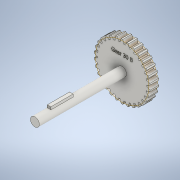
# Autodesk Inventor part: Spur_Gear12
Saved by Autodesk Inventor 2021 (Build 250183000, 183)
## iProperties
Created: 2021-04-10
Part Number: Spur_Gear12
Material: Steel
Document SubType Name: Modeling
Designer: Nabeel Azafer
Categories: <?xml version="1.0" encoding="UTF-16"?> <MemberInstance><Categories><FamilyTemplate><FamilyTemplateParameter ValueType="xs:double" Id="1" ObjectReferenceKey="da_z" ObjectType="kUserParameterObject"/><FamilyTemplateParameter ValueType="xs:double" Id="2" ObjectReferenceKey="da_b" ObjectType="kUserParameterObject"/><FamilyTemplateParameter ValueType="xs:double" Id="3" ObjectReferenceKey="da_beta" ObjectType="kUserParameterObject"/><FamilyTemplateParameter ValueType="xs:double" Id="4" ObjectReferenceKey="da_da" ObjectType="kUserParameterObject"/><FamilyTemplateParameter ValueType="xs:double" Id="5" ObjectReferenceKey="da_aw" ObjectType="kUserParameterObject"/><FamilyTemplateParameter ValueType="xs:string" Id="6" ObjectReferenceKey="EAIAABAAAACIAQAAAAAAAIAAAAAAAAAA" ObjectType="83910656" SubObjectId="SurfaceGeometry"/></FamilyTemplate><ParamToTemplateMap><ParamToTemplate CategoryParameter="//CategoryParameter[@InternalName='046C89C9-8512-4d59-83FE-43B91F4F132A']" TemplateParameter="1"/><ParamToTemplate CategoryParameter="//CategoryParameter[@InternalName='2552DF32-E462-4b46-AEBF-C6C7768E72AC']" TemplateParameter="2"/><ParamToTemplate CategoryParameter="//CategoryParameter[@InternalName='C9EE641D-15FC-4fae-A226-E94C4372FDD7']" TemplateParameter="3"/><ParamToTemplate><ParamToTemplate CategoryParameter="//CategoryParameter[@InternalName='00B6519A-459B-49c7-AD84-2E56D39A5744']" ConstantValue="0.000000"/></ParamToTemplate><ParamToTemplate><ParamToTemplate CategoryParameter="//CategoryParameter[@InternalName='04B31F0E-C7A6-4894-AA32-9629BEFACF47']" ConstantValue="0.800000"/></ParamToTemplate><ParamToTemplate><ParamToTemplate CategoryParameter="//CategoryParameter[@InternalName='43CBEC2E-7847-49e7-A936-2F7889FCB2D9']" ConstantValue="0.350000"/></ParamToTemplate><ParamToTemplate><ParamToTemplate CategoryParameter="//CategoryParameter[@InternalName='B1EFC894-105D-4ebd-86BF-FA20ED196853']" ConstantValue="0.500000"/></ParamToTemplate><ParamToTemplate><ParamToTemplate CategoryParameter="//CategoryParameter[@InternalName='51175063-3D10-4879-93E8-6246FE8B403D']" ConstantValue="2060000000.000000"/></ParamToTemplate><ParamToTemplate><ParamToTemplate CategoryParameter="//CategoryParameter[@InternalName='A3A52E27-4454-46a9-B0BD-C932399B70AF']" ConstantValue="0.300000"/></ParamToTemplate><ParamToTemplate><ParamToTemplate CategoryParameter="//CategoryParameter[@InternalName='91B76062-C214-41d9-B1B9-14D2AB99603D']" ConstantValue="0.100000"/></ParamToTemplate><ParamToTemplate><ParamToTemplate CategoryParameter="//CategoryParameter[@InternalName='374E806E-8B8A-4dda-A9AA-1039D6500AD2']" ConstantValue="10.000000"/></ParamToTemplate><ParamToTemplate><ParamToTemplate CategoryParameter="//CategoryParameter[@InternalName='2D373A89-B862-43d6-8D0B-0CBF12AB9F6C']" ConstantValue="0.349066"/></ParamToTemplate><ParamToTemplate CategoryParameter="//CategoryParameter[@InternalName='37777632-D6A2-4fac-9D53-DB8ACD95C989']" TemplateParameter="4"/><ParamToTemplate CategoryParameter="//CategoryParameter[@InternalName='FD1017F1-B727-4f7e-9707-0F86F1FF9423']" TemplateParameter="5"/><ParamToTemplate><ParamToTemplate CategoryParameter="//CategoryParameter[@InternalName='9E1B4470-B2D3-4ff1-B813-535BB4CDF51A']" ConstantValue="3520000.000000"/></ParamToTemplate><ParamToTemplate><ParamToTemplate CategoryParameter="//CategoryParameter[@InternalName='F8452263-BFF6-458c-9FB1-07C4B99E95CD']" ConstantValue="11400000.000000"/></ParamToTemplate><ParamToTemplate><ParamToTemplate CategoryParameter="//CategoryParameter[@InternalName='3E3BB259-FD49-497f-8171-6EBC954A3479']" ConstantValue="2.000000"/></ParamToTemplate><ParamToTemplate CategoryParameter="//CategoryParameter[@InternalName='27C3BAF2-7550-4e4b-AE2C-0DB134B7D9B7']" TemplateParameter="6"/></ParamToTemplateMap><Category DisplayName="Gear" InternalName="DC85795E-93AB-48d5-8EEE-5A27447B64BD" Mnemonic="Gear"><CategoryParameter DisplayName="z" InternalName="046C89C9-8512-4d59-83FE-43B91F4F132A" Mnemonic="z"/><CategoryParameter DisplayName="b" InternalName="2552DF32-E462-4b46-AEBF-C6C7768E72AC" Mnemonic="b"/><CategoryParameter DisplayName="||b|" InternalName="C9EE641D-15FC-4fae-A226-E94C4372FDD7" Mnemonic="beta"/><CategoryParameter DisplayName="x" InternalName="00B6519A-459B-49c7-AD84-2E56D39A5744" Mnemonic="x"/><CategoryParameter DisplayName="a*" InternalName="04B31F0E-C7A6-4894-AA32-9629BEFACF47" Mnemonic="a"/><CategoryParameter DisplayName="c*" InternalName="43CBEC2E-7847-49e7-A936-2F7889FCB2D9" Mnemonic="c"/><CategoryParameter DisplayName="r|.f|*" InternalName="B1EFC894-105D-4ebd-86BF-FA20ED196853" Mnemonic="rf"/><CategoryParameter DisplayName="E" InternalName="51175063-3D10-4879-93E8-6246FE8B403D" Mnemonic="E"/><CategoryParameter DisplayName="||m|" InternalName="A3A52E27-4454-46a9-B0BD-C932399B70AF" Mnemonic="mi"/><Category DisplayName="SpurGear" InternalName="26C5A22E-A91E-4dfd-A3B3-23CCAFAE1764" Mnemonic="SpurGear"><CategoryParameter DisplayName="m" InternalName="91B76062-C214-41d9-B1B9-14D2AB99603D" Mnemonic="m"/><CategoryParameter DisplayName="P" InternalName="374E806E-8B8A-4dda-A9AA-1039D6500AD2" Mnemonic="PP"/><CategoryParameter DisplayName="||a|" InternalName="2D373A89-B862-43d6-8D0B-0CBF12AB9F6C" Mnemonic="alpha"/><CategoryParameter DisplayName="d|.a|" InternalName="37777632-D6A2-4fac-9D53-DB8ACD95C989" Mnemonic="da"/><CategoryParameter DisplayName="a|.w|" InternalName="FD1017F1-B727-4f7e-9707-0F86F1FF9423" Mnemonic="aw"/><CategoryParameter DisplayName="||s||.Flim|" InternalName="9E1B4470-B2D3-4ff1-B813-535BB4CDF51A" Mnemonic="sFlim"/><CategoryParameter DisplayName="||s||.Hlim|" InternalName="F8452263-BFF6-458c-9FB1-07C4B99E95CD" Mnemonic="sHlim"/><CategoryParameter DisplayName="type" InternalName="3E3BB259-FD49-497f-8171-6EBC954A3479" Mnemonic="type"/><CategoryParameter DisplayName="PitchDiameter" InternalName="27C3BAF2-7550-4e4b-AE2C-0DB134B7D9B7" Mnemonic="IDS_PITCHDIAM"/></Category></Category></Categories></MemberInstance>
Density: 7.85 g/cm^3
Appearance: Steel
Mass: 43.2565 g
Surface Area: 28.3538 cm^2
Volume: 5.51038 cm^3
Author: Nabeel Azafer
Autodesk Inventor part; units mm, degrees
note: some values were not read from the file. Chosen so that the rebuilt part matches the saved one: direction of "Emboss1".
sketch "Sketch1" plane through (0, 0, 0) normal (0, 0, 1) x (1, 0, 0)
  circle A0 centre (0, 0) radius 15.8
  dimension "d0" = 31.6
  constraints: 1 centre point
  measures "d0" diameter of A0
extrude "Extrusion1" add sketch "Sketch1" along normal blind 5
ref_plane "Work Plane2" through (0, 0, 2.5) normal (0, 0, 1) x (1, 0, 0)
sketch "Sketch2" plane through (0, 0, 0) normal (0, 0, -1) x (-1, 0, 0)
  circle A0 centre (0, 0) radius 15.8 projected
  circle A1 centre (0, 0) radius 15
  dimension "d3" = 30
  constraints: 1 centre point, 1 coincident
  measures "d3" diameter of A1
surface extrude "Pitch Diameter" sketch "Sketch2" against normal through all shown yes curves A1
ref_plane "Work Plane8" through (0, 0, 0) normal (0.9945219, 0.1045285, 0) x (0, 0, 1)
ref_plane "Work Plane9" through (0, 0, 0) normal (1, 0, 0) x (0, 1, 0)
spur gear teeth "Spur Gear" teeth 30 pitch diameter 30 tip diameter 31.6 root diameter 27.7 face width 8 start plane through (0, 0, 0) normal (0, 0, -1) x (-1, 0, 0)
sketch "Sketch5" plane through (0, 0, 5) normal (0, 0, 1) x (1, 0, 0)
  circle A0 centre (0, 0) radius 2.5
  dimension "d63" = 5
  constraints: 1 centre point, 1 coincident
  measures "d63" diameter of A0
extrude "Extrusion3" add sketch "Sketch5" along normal blind 41
sketch "Sketch6" plane through (0, 0, 46) normal (0, 0, 1) x (1, 0, 0)
  point P0 (0, 0)
sketch "Sketch7" plane through (0, 0, 46) normal (0, 0, 1) x (1, 0, 0)
  circle A0 centre (0, 0) radius 2.5 projected
  line L0 (-1, 2.2913) -> (1, 2.2913)
  line L1 (1, 2.2913) -> (1, 3.7913)
  line L2 (1, 3.7913) -> (-1, 3.7913)
  line L3 (-1, 3.7913) -> (-1, 2.2913)
  dimension "d70" = 2
  dimension "d71" = 1.5
  constraints: 8 end point, 2 parallel, 1 horizontal, 1 perpendicular, 2 other
  measures "d70" distance of L2.end L1.end
  measures "d71" distance of L1.end L0.end
extrude "Extrusion4" add sketch "Sketch7" against normal blind 12.5 contours L0 A0 | A0 L3 L2 L1 picked at (-0.1703, 2.3433)
sketch "Sketch8" plane through (0, 0, 0) normal (0, 0, -1) x (-1, 0, 0)
  circle A0 centre (0, 0) radius 2.5
  dimension "d74" = 5
  constraints: 1 centre point, 1 coincident
  measures "d74" diameter of A0
extrude "Extrusion5" add sketch "Sketch8" along normal blind 8
sketch "Sketch9" plane through (0, 0, 46) normal (0, 0, 1) x (1, 0, 0)
  circle A0 centre (0, 0) radius 2.5
  constraints: 1 centre point, 1 coincident
extrude "Extrusion6" add sketch "Sketch9" along normal blind 8
sketch "Sketch10" plane through (0, 0, 5) normal (0, 0, 1) x (1, 0, 0)
  line L0 (-6.024, 9.3702) -> (6.4531, 9.3702) construction
  line L1 (6.4531, 9.3702) -> (6.4531, 4.357) construction
  line L2 (6.4531, 4.357) -> (-6.024, 4.357) construction
  line L3 (-6.024, 4.357) -> (-6.024, 9.3702) construction
  spline S0 degree 2 poles (-4.9835, 7.2891) (-5.1958, 7.2891) (-5.5475, 7.4188) (-5.674, 7.5501) knots 0 0 0 1 2 2 2
  spline S1 degree 2 poles (-5.674, 7.5501) (-5.8004, 7.683) (-5.9349, 8.0752) (-5.9349, 8.3296) knots 0 0 0 1 2 2 2
  spline S2 degree 2 poles (-5.9349, 8.3296) (-5.9349, 8.5711) (-5.7988, 8.9536) (-5.6723, 9.0898) knots 0 0 0 1 2 2 2
  spline S3 degree 2 poles (-5.6723, 9.0898) (-5.5508, 9.2211) (-5.1942, 9.3637) (-4.9819, 9.3637) knots 0 0 0 1 2 2 2
  spline S4 degree 2 poles (-4.9819, 9.3637) (-4.8798, 9.3637) (-4.695, 9.3345) (-4.6107, 9.3086) knots 0 0 0 1 2 2 2
  spline S5 degree 2 poles (-4.6107, 9.3086) (-4.5427, 9.2891) (-4.3774, 9.2178) (-4.3271, 9.1919) knots 0 0 0 1 2 2 2
  line L4 (-4.3271, 9.1919) -> (-4.3271, 8.871)
  line L5 (-4.3271, 8.871) -> (-4.3498, 8.871)
  spline S6 degree 2 poles (-4.3498, 8.871) (-4.4, 8.9147) (-4.5054, 8.9941) (-4.6026, 9.0395) knots 0 0 0 1 2 2 2
  spline S7 degree 2 poles (-4.6026, 9.0395) (-4.6837, 9.08) (-4.8928, 9.1335) (-5.0127, 9.1335) knots 0 0 0 1 2 2 2
  spline S8 degree 2 poles (-5.0127, 9.1335) (-5.3012, 9.1335) (-5.6577, 8.6992) (-5.6577, 8.3377) knots 0 0 0 1 2 2 2
  spline S9 degree 2 poles (-5.6577, 8.3377) (-5.6577, 8.1368) (-5.5637, 7.8353) (-5.4746, 7.7316) knots 0 0 0 1 2 2 2
  spline S10 degree 2 poles (-5.4746, 7.7316) (-5.3887, 7.6279) (-5.1456, 7.5193) (-4.9932, 7.5193) knots 0 0 0 1 2 2 2
  spline S11 degree 2 poles (-4.9932, 7.5193) (-4.8814, 7.5193) (-4.6577, 7.5517) (-4.5816, 7.5841) knots 0 0 0 1 2 2 2
  line L6 (-4.5816, 7.5841) -> (-4.5816, 8.1011)
  line L7 (-4.5816, 8.1011) -> (-5.0451, 8.1011)
  line L8 (-5.0451, 8.1011) -> (-5.0451, 8.3345)
  line L9 (-5.0451, 8.3345) -> (-4.319, 8.3345)
  line L10 (-4.319, 8.3345) -> (-4.319, 7.4609)
  spline S12 degree 2 poles (-4.319, 7.4609) (-4.3693, 7.4382) (-4.5411, 7.3685) (-4.614, 7.3475) knots 0 0 0 1 2 2 2
  spline S13 degree 2 poles (-4.614, 7.3475) (-4.7129, 7.3183) (-4.8717, 7.2891) (-4.9835, 7.2891) knots 0 0 0 1 2 2 2
  spline S14 degree 2 poles (-3.353, 7.294) (-3.7129, 7.294) (-4.1083, 7.6976) (-4.1083, 8.0703) knots 0 0 0 1 2 2 2
  spline S15 degree 2 poles (-4.1083, 8.0703) (-4.1083, 8.4366) (-3.7242, 8.871) (-3.4146, 8.871) knots 0 0 0 1 2 2 2
  spline S16 degree 2 poles (-3.4146, 8.871) (-3.2752, 8.871) (-3.0597, 8.7899) (-2.9803, 8.704) knots 0 0 0 1 2 2 2
  spline S17 degree 2 poles (-2.9803, 8.704) (-2.8992, 8.6181) (-2.8133, 8.3702) (-2.8133, 8.1903) knots 0 0 0 1 2 2 2
  line L11 (-2.8133, 8.1903) -> (-2.8133, 8.0525)
  line L12 (-2.8133, 8.0525) -> (-3.8522, 8.0525)
  spline S18 degree 2 poles (-3.8522, 8.0525) (-3.8522, 7.7916) (-3.5897, 7.5144) (-3.3563, 7.5144) knots 0 0 0 1 2 2 2
  spline S19 degree 2 poles (-3.3563, 7.5144) (-3.2736, 7.5144) (-3.1132, 7.5517) (-3.0483, 7.5809) knots 0 0 0 1 2 2 2
  spline S20 degree 2 poles (-3.0483, 7.5809) (-2.9803, 7.6133) (-2.8863, 7.67) (-2.8555, 7.6959) knots 0 0 0 1 2 2 2
  line L13 (-2.8555, 7.6959) -> (-2.8409, 7.6959)
  line L14 (-2.8409, 7.6959) -> (-2.8409, 7.4204)
  spline S21 degree 2 poles (-2.8409, 7.4204) (-2.8847, 7.4026) (-3.0176, 7.3507) (-3.0694, 7.3361) knots 0 0 0 1 2 2 2
  spline S22 degree 2 poles (-3.0694, 7.3361) (-3.1423, 7.3151) (-3.2623, 7.294) (-3.353, 7.294) knots 0 0 0 1 2 2 2
  spline S23 degree 2 poles (-3.0597, 8.2454) (-3.0629, 8.3475) (-3.1051, 8.4966) (-3.1456, 8.5468) knots 0 0 0 1 2 2 2
  spline S24 degree 2 poles (-3.1456, 8.5468) (-3.1894, 8.6035) (-3.3271, 8.6635) (-3.4292, 8.6635) knots 0 0 0 1 2 2 2
  spline S25 degree 2 poles (-3.4292, 8.6635) (-3.5297, 8.6635) (-3.6707, 8.6035) (-3.7291, 8.5452) knots 0 0 0 1 2 2 2
  spline S26 degree 2 poles (-3.7291, 8.5452) (-3.7858, 8.4852) (-3.8441, 8.341) (-3.8522, 8.2454) knots 0 0 0 1 2 2 2
  line L15 (-3.8522, 8.2454) -> (-3.0597, 8.2454)
  spline S27 degree 2 poles (-1.721, 7.4869) (-1.7517, 7.4642) (-1.8555, 7.3831) (-1.9041, 7.3588) knots 0 0 0 1 2 2 2
  spline S28 degree 2 poles (-1.9041, 7.3588) (-1.9705, 7.3232) (-2.0953, 7.2859) (-2.2088, 7.2859) knots 0 0 0 1 2 2 2
  spline S29 degree 2 poles (-2.2088, 7.2859) (-2.3012, 7.2859) (-2.4681, 7.3556) (-2.5313, 7.4188) knots 0 0 0 1 2 2 2
  spline S30 degree 2 poles (-2.5313, 7.4188) (-2.5913, 7.4804) (-2.6642, 7.6619) (-2.6642, 7.7624) knots 0 0 0 1 2 2 2
  spline S31 degree 2 poles (-2.6642, 7.7624) (-2.6642, 7.918) (-2.5329, 8.1384) (-2.3903, 8.2016) knots 0 0 0 1 2 2 2
  spline S32 degree 2 poles (-2.3903, 8.2016) (-2.2639, 8.26) (-1.9203, 8.3037) (-1.721, 8.3151) knots 0 0 0 1 2 2 2
  line L16 (-1.721, 8.3151) -> (-1.721, 8.3637)
  spline S33 degree 2 poles (-1.721, 8.3637) (-1.721, 8.4512) (-1.7744, 8.5598) (-1.8231, 8.5906) knots 0 0 0 1 2 2 2
  spline S34 degree 2 poles (-1.8231, 8.5906) (-1.8717, 8.6214) (-2.0111, 8.6408) (-2.0856, 8.6408) knots 0 0 0 1 2 2 2
  spline S35 degree 2 poles (-2.0856, 8.6408) (-2.1731, 8.6408) (-2.4098, 8.589) (-2.5281, 8.5387) knots 0 0 0 1 2 2 2
  line L17 (-2.5281, 8.5387) -> (-2.5427, 8.5387)
  line L18 (-2.5427, 8.5387) -> (-2.5427, 8.7964)
  spline S36 degree 2 poles (-2.5427, 8.7964) (-2.473, 8.8159) (-2.212, 8.8645) (-2.084, 8.8645) knots 0 0 0 1 2 2 2
  spline S37 degree 2 poles (-2.084, 8.8645) (-1.9284, 8.8645) (-1.7161, 8.8159) (-1.6318, 8.7527) knots 0 0 0 1 2 2 2
  spline S38 degree 2 poles (-1.6318, 8.7527) (-1.5492, 8.6911) (-1.4681, 8.495) (-1.4681, 8.354) knots 0 0 0 1 2 2 2
  line L19 (-1.4681, 8.354) -> (-1.4681, 7.328)
  line L20 (-1.4681, 7.328) -> (-1.721, 7.328)
  line L21 (-1.721, 7.328) -> (-1.721, 7.4869)
  line L22 (-1.721, 7.6976) -> (-1.721, 8.1141)
  spline S39 degree 2 poles (-1.721, 8.1141) (-1.8117, 8.106) (-2.0856, 8.0784) (-2.1715, 8.0525) knots 0 0 0 1 2 2 2
  spline S40 degree 2 poles (-2.1715, 8.0525) (-2.272, 8.0217) (-2.4033, 7.8937) (-2.4033, 7.7802) knots 0 0 0 1 2 2 2
  spline S41 degree 2 poles (-2.4033, 7.7802) (-2.4033, 7.6506) (-2.2574, 7.5193) (-2.118, 7.5193) knots 0 0 0 1 2 2 2
  spline S42 degree 2 poles (-2.118, 7.5193) (-1.9997, 7.5193) (-1.8052, 7.6214) (-1.721, 7.6976) knots 0 0 0 1 2 2 2
  line L23 (-0.3174, 8.5582) -> (-0.3304, 8.5582)
  spline S43 degree 2 poles (-0.3304, 8.5582) (-0.3595, 8.5663) (-0.4227, 8.5695) (-0.4665, 8.5695) knots 0 0 0 1 2 2 2
  spline S44 degree 2 poles (-0.4665, 8.5695) (-0.5686, 8.5695) (-0.7696, 8.4804) (-0.8603, 8.3929) knots 0 0 0 1 2 2 2
  line L24 (-0.8603, 8.3929) -> (-0.8603, 7.328)
  line L25 (-0.8603, 7.328) -> (-1.1132, 7.328)
  line L26 (-1.1132, 7.328) -> (-1.1132, 8.8288)
  line L27 (-1.1132, 8.8288) -> (-0.8603, 8.8288)
  line L28 (-0.8603, 8.8288) -> (-0.8603, 8.6052)
  spline S45 degree 2 poles (-0.8603, 8.6052) (-0.7226, 8.7283) (-0.5167, 8.8288) (-0.4195, 8.8288) knots 0 0 0 1 2 2 2
  spline S46 degree 2 poles (-0.4195, 8.8288) (-0.3806, 8.8288) (-0.3417, 8.8256) (-0.3174, 8.8207) knots 0 0 0 1 2 2 2
  line L29 (-0.3174, 8.8207) -> (-0.3174, 8.5582)
  spline S47 degree 2 poles (1.2401, 9.1384) (1.1672, 9.1384) (1.023, 9.1027) (0.9533, 9.0752) knots 0 0 0 1 2 2 2
  spline S48 degree 2 poles (0.9533, 9.0752) (0.8884, 9.0476) (0.7928, 8.9893) (0.7555, 8.9634) knots 0 0 0 1 2 2 2
  line L30 (0.7555, 8.9634) -> (0.7393, 8.9634)
  line L31 (0.7393, 8.9634) -> (0.7393, 9.247)
  spline S49 degree 2 poles (0.7393, 9.247) (0.8269, 9.294) (1.1267, 9.3702) (1.2612, 9.3702) knots 0 0 0 1 2 2 2
  spline S50 degree 2 poles (1.2612, 9.3702) (1.3974, 9.3702) (1.6, 9.3151) (1.6826, 9.2567) knots 0 0 0 1 2 2 2
  spline S51 degree 2 poles (1.6826, 9.2567) (1.7701, 9.1935) (1.8609, 9.0104) (1.8609, 8.8872) knots 0 0 0 1 2 2 2
  spline S52 degree 2 poles (1.8609, 8.8872) (1.8609, 8.7219) (1.6437, 8.4723) (1.4914, 8.4399) knots 0 0 0 1 2 2 2
  line L32 (1.4914, 8.4399) -> (1.4914, 8.4204)
  spline S53 degree 2 poles (1.4914, 8.4204) (1.5546, 8.4074) (1.6988, 8.3491) (1.7604, 8.2907) knots 0 0 0 1 2 2 2
  spline S54 degree 2 poles (1.7604, 8.2907) (1.822, 8.234) (1.8998, 8.0525) (1.8998, 7.9212) knots 0 0 0 1 2 2 2
  spline S55 degree 2 poles (1.8998, 7.9212) (1.8998, 7.7867) (1.8074, 7.5582) (1.7231, 7.4706) knots 0 0 0 1 2 2 2
  spline S56 degree 2 poles (1.7231, 7.4706) (1.6356, 7.3799) (1.3876, 7.2859) (1.2304, 7.2859) knots 0 0 0 1 2 2 2
  spline S57 degree 2 poles (1.2304, 7.2859) (1.0797, 7.2859) (0.7847, 7.3588) (0.6842, 7.4091) knots 0 0 0 1 2 2 2
  line L33 (0.6842, 7.4091) -> (0.6842, 7.6927)
  line L34 (0.6842, 7.6927) -> (0.7037, 7.6927)
  spline S58 degree 2 poles (0.7037, 7.6927) (0.788, 7.6311) (1.0732, 7.5177) (1.2142, 7.5177) knots 0 0 0 1 2 2 2
  spline S59 degree 2 poles (1.2142, 7.5177) (1.2969, 7.5177) (1.4622, 7.5695) (1.5173, 7.6295) knots 0 0 0 1 2 2 2
  spline S60 degree 2 poles (1.5173, 7.6295) (1.5708, 7.6894) (1.6275, 7.8321) (1.6275, 7.9407) knots 0 0 0 1 2 2 2
  spline S61 degree 2 poles (1.6275, 7.9407) (1.6275, 8.0493) (1.5643, 8.1903) (1.5076, 8.2308) knots 0 0 0 1 2 2 2
  spline S62 degree 2 poles (1.5076, 8.2308) (1.4508, 8.2713) (1.2969, 8.3021) (1.2061, 8.3021) knots 0 0 0 1 2 2 2
  line L35 (1.2061, 8.3021) -> (1.0927, 8.3021)
  line L36 (1.0927, 8.3021) -> (1.0927, 8.5241)
  line L37 (1.0927, 8.5241) -> (1.1818, 8.5241)
  spline S63 degree 2 poles (1.1818, 8.5241) (1.3617, 8.5241) (1.5886, 8.6959) (1.5886, 8.8596) knots 0 0 0 1 2 2 2
  spline S64 degree 2 poles (1.5886, 8.8596) (1.5886, 8.9358) (1.5303, 9.0444) (1.4833, 9.0768) knots 0 0 0 1 2 2 2
  spline S65 degree 2 poles (1.4833, 9.0768) (1.433, 9.1108) (1.3098, 9.1384) (1.2401, 9.1384) knots 0 0 0 1 2 2 2
  spline S66 degree 2 poles (3.446, 8.328) (3.446, 7.7899) (3.1332, 7.2859) (2.8074, 7.2859) knots 0 0 0 1 2 2 2
  spline S67 degree 2 poles (2.8074, 7.2859) (2.4768, 7.2859) (2.1672, 7.7997) (2.1672, 8.3264) knots 0 0 0 1 2 2 2
  spline S68 degree 2 poles (2.1672, 8.3264) (2.1672, 8.8677) (2.48, 9.3685) (2.8074, 9.3685) knots 0 0 0 1 2 2 2
  spline S69 degree 2 poles (2.8074, 9.3685) (3.1364, 9.3685) (3.446, 8.8499) (3.446, 8.328) knots 0 0 0 1 2 2 2
  spline S70 degree 2 poles (3.1024, 7.7186) (3.1413, 7.8175) (3.1737, 8.1222) (3.1737, 8.328) knots 0 0 0 1 2 2 2
  spline S71 degree 2 poles (3.1737, 8.328) (3.1737, 8.5339) (3.1413, 8.8369) (3.1008, 8.939) knots 0 0 0 1 2 2 2
  spline S72 degree 2 poles (3.1008, 8.939) (3.0602, 9.0412) (2.9192, 9.1465) (2.8074, 9.1465) knots 0 0 0 1 2 2 2
  spline S73 degree 2 poles (2.8074, 9.1465) (2.6956, 9.1465) (2.5513, 9.0412) (2.5092, 8.9358) knots 0 0 0 1 2 2 2
  spline S74 degree 2 poles (2.5092, 8.9358) (2.4687, 8.8337) (2.4395, 8.5225) (2.4395, 8.3264) knots 0 0 0 1 2 2 2
  spline S75 degree 2 poles (2.4395, 8.3264) (2.4395, 8.1157) (2.4654, 7.8337) (2.5076, 7.7235) knots 0 0 0 1 2 2 2
  spline S76 degree 2 poles (2.5076, 7.7235) (2.5465, 7.6198) (2.6907, 7.5079) (2.8074, 7.5079) knots 0 0 0 1 2 2 2
  spline S77 degree 2 poles (2.8074, 7.5079) (2.9176, 7.5079) (3.0619, 7.6133) (3.1024, 7.7186) knots 0 0 0 1 2 2 2
  spline S78 degree 2 poles (5.9743, 7.9423) (5.9743, 7.7932) (5.8609, 7.5647) (5.7669, 7.4901) knots 0 0 0 1 2 2 2
  spline S79 degree 2 poles (5.7669, 7.4901) (5.6534, 7.4026) (5.3957, 7.328) (5.1915, 7.328) knots 0 0 0 1 2 2 2
  line L38 (5.1915, 7.328) -> (4.6178, 7.328)
  line L39 (4.6178, 7.328) -> (4.6178, 9.328)
  line L40 (4.6178, 9.328) -> (5.1478, 9.328)
  spline S80 degree 2 poles (5.1478, 9.328) (5.3617, 9.328) (5.5756, 9.3005) (5.6729, 9.247) knots 0 0 0 1 2 2 2
  spline S81 degree 2 poles (5.6729, 9.247) (5.7815, 9.1903) (5.8803, 9.0039) (5.8803, 8.8775) knots 0 0 0 1 2 2 2
  spline S82 degree 2 poles (5.8803, 8.8775) (5.8803, 8.7365) (5.7312, 8.5128) (5.6, 8.4496) knots 0 0 0 1 2 2 2
  line L41 (5.6, 8.4496) -> (5.6, 8.4399)
  spline S83 degree 2 poles (5.6, 8.4399) (5.7782, 8.3912) (5.9743, 8.1335) (5.9743, 7.9423) knots 0 0 0 1 2 2 2
  spline S84 degree 2 poles (5.6972, 7.9309) (5.6972, 8.0444) (5.6324, 8.1903) (5.5351, 8.2421) knots 0 0 0 1 2 2 2
  spline S85 degree 2 poles (5.5351, 8.2421) (5.4719, 8.2745) (5.3228, 8.294) (5.185, 8.294) knots 0 0 0 1 2 2 2
  line L42 (5.185, 8.294) -> (4.8836, 8.294)
  line L43 (4.8836, 8.294) -> (4.8836, 7.5549)
  line L44 (4.8836, 7.5549) -> (5.0991, 7.5549)
  spline S86 degree 2 poles (5.0991, 7.5549) (5.2742, 7.5549) (5.4752, 7.5873) (5.553, 7.6392) knots 0 0 0 1 2 2 2
  spline S87 degree 2 poles (5.553, 7.6392) (5.6275, 7.6927) (5.6972, 7.8256) (5.6972, 7.9309) knots 0 0 0 1 2 2 2
  spline S88 degree 2 poles (5.6032, 8.8402) (5.6032, 8.9115) (5.5546, 9.0185) (5.5011, 9.0493) knots 0 0 0 1 2 2 2
  spline S89 degree 2 poles (5.5011, 9.0493) (5.4363, 9.0849) (5.279, 9.1011) (5.138, 9.1011) knots 0 0 0 1 2 2 2
  line L45 (5.138, 9.1011) -> (4.8836, 9.1011)
  line L46 (4.8836, 9.1011) -> (4.8836, 8.516)
  line L47 (4.8836, 8.516) -> (5.185, 8.516)
  spline S90 degree 2 poles (5.185, 8.516) (5.3098, 8.516) (5.4282, 8.542) (5.4914, 8.5825) knots 0 0 0 1 2 2 2
  spline S91 degree 2 poles (5.4914, 8.5825) (5.553, 8.6214) (5.6032, 8.7462) (5.6032, 8.8402) knots 0 0 0 1 2 2 2
  point P0 (0, 0)
  constraints: 2 other
emboss "Emboss1" sketch "Sketch10" operation cut depth 1 direction (0, 0, -1)
equation "\"d0\" = da_da"
equation "\"d3\" = da_d"
equation "\"d16\" = da_aw"
equation "\"d43\" = da_aw"
equation "\"d46\" = da_aw"
equation "\"da_da\" = 31.6"
equation "\"da_d\" = 30"
equation "\"da_aw\" = 22.5"
body "Solid1"
body "Srf1"
